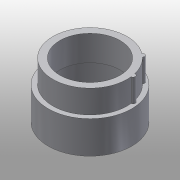
# Autodesk Inventor part: 500-136
Saved by Autodesk Inventor 2016 (Build 200138000, 138)
## iProperties
Created: 2015-04-18
Part Number: 500-136
Material: ABS Plastic
Document SubType Name: Modeling
Designer: Station9
Density: 1.06 g/cm^3
Appearance: Smooth - White
Mass: 0.79886 g
Surface Area: 14.4801 cm^2
Volume: 0.753642 cm^3
Author: Station9
Autodesk Inventor part; units mm, degrees
ref_plane "YZ Plane" through (0, 0, 0) normal (1, 0, 0) x (0, 1, 0)
ref_plane "XZ Plane" through (0, 0, 0) normal (0, 1, 0) x (-1, 0, 0)
ref_plane "XY Plane" through (0, 0, 0) normal (0, 0, 1) x (1, 0, 0)
sketch "Sketch4" plane through (0, 0, 0) normal (0, 1, 0) x (-1, 0, 0)
  line L0 (0, 0) -> (0, -19.6155)
  line L1 (-8, 0) -> (-6.5, 0)
  line L2 (-6.5, 0) -> (-6.5, -5)
  line L3 (-8, -5) -> (-8, 0)
  line L4 (-8, -5) -> (-9, -5)
  line L5 (-9, -5) -> (-9, -12)
  line L6 (-9, -12) -> (-8, -12)
  line L7 (-9, -5) -> (-8, -5)
  line L8 (-9, -9.8345) -> (-9, -5)
  line L9 (-8, -12) -> (-8, -5.5)
  line L10 (-8, -5.5) -> (-6.5, -5.5)
  line L11 (-6.5, -5.5) -> (-6.5, -5)
  dimension "d9" = 18
  dimension "d10" = 16
  dimension "d13" = 7
  dimension "d14" = 0
  dimension "d15" = 5
  dimension "d16" = 6.5
  dimension "d17" = 13
  dimension "d18" = 16
  constraints: 24 end point, 4 horizontal, 3 vertical, 2 parallel, 2 perpendicular
  measures "d9" diameter of L5 L0
  measures "d10" diameter of L3 L0
  measures "d13" distance of L4.end L5.end
  measures "d14" distance from line of L0.start L1
  measures "d15" distance of L3.start L1.start
  measures "d16" distance of L6.end L9.end
  measures "d17" diameter of L2 L0
  measures "d18" diameter of L9 L0
revolve "Revolution1" add sketch "Sketch4" angle 360 about axis through (0, 0, 0) along (0, 0, -1)
sketch "Sketch5" plane through (0, 0, 0) normal (0, 0, 1) x (1, 0, 0)
  circle A0 centre (0, 0) radius 8 projected
  circle A1 centre (0, 0) radius 6.5 projected
  line L0 (0, 0) -> (7.8785, 1.3892)
  circle A2 centre (0, 0) radius 8 projected
  line L1 (0, 0) -> (5.4955, 0)
  line L2 (0, 0) -> (5.1423, 6.1284)
  circle A3 centre (5.1423, 6.1284) radius 0.5
  circle A4 centre (7.8785, 1.3892) radius 0.5
  dimension "d20" = 10
  dimension "d21" = 40
  dimension "d22" = 1
  dimension "d23" = 1
  constraints: 6 end point, 4 point on circle, 2 centre point, 2 coincident, 1 horizontal
  measures "d20" angle of L0 L1
  measures "d21" angle of L2 L0
  measures "d22" diameter of A3
  measures "d23" diameter of A4
extrude "Extrusion4" add sketch "Sketch5" against normal up to surface (5 mm away) contours A4 L0 A0 | A0 A4 | A3 A0 | A0 L2 A3 | L0 A4 A0 | A0 A3 L2
body "Solid2"
